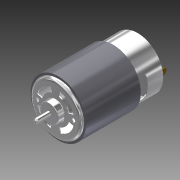
# Autodesk Inventor part: RS-550
Saved by Autodesk Inventor 2015 SP1 (Build 190203100, 203)
## iProperties
Category: Motors
Company: Autodesk, Inc.
Shininess: 64.0
Length Units: 11269
Angle Units: 11279
Time Units: 11290
Mass Units: 11283
Length Display Precision: 3
Angle Display Precision: 2
Compacted: True
Part Number: RS-550
Document SubType Name: Modeling
Created: 2014-12-12
Material: Steel, Mild
Project: FIRST
Catalog Web Link: http://banebots.com/pc/p/M5-RS550-12
Vendor: BaneBots
Density: 40.6947 g/cm^3
Description: Motor - BaneBots RS-550
Mass: 221 g
Surface Area: 167.862 cm^2
Volume: 12.5148 cm^3
Appearance: Chrome - Polished
Density: 0.0
Volumn: 0.0
Area: 0.0
PropertySet Name: Model Information
Control State: 0
Master: False
Checked Out: False
Title: Motor - BaneBots RS-550
Author: Autodesk, Inc.
Autodesk Inventor part; units mm, degrees
sketch "Sketch1" plane through (0, 0, 0) normal (0, 0, 1) x (1, 0, 0)
  circle A0 centre (0, 0) radius 17.75
  dimension "d0" = 35.5
  constraints: 2 coincident, 1 centre point, 2 other
  measures "d0" diameter of A0
extrude "Extrusion1" add sketch "Sketch1" along normal mid plane 57
fillet "Fillet1" radius 2 1 edges at (-17.75, 0, 28.5)
shell "Shell1" thickness 0.62 removed faces 1 at (3.0438, 4.2648, -28.5)
sketch "Sketch2" plane through (0, 0, 28.5) normal (0, 0, 1) x (1, 0, 0)
  circle A0 centre (0, 0) radius 15.75 projected
  circle A1 centre (0, 0) radius 6.5
  dimension "d5" = 13
  constraints: 1 centre point, 1 coincident, 1 concentric
  measures "d5" diameter of A1
extrude "Extrusion2" add sketch "Sketch2" along normal blind 4.5 contours A1
fillet "Fillet2" radius 0.5 2 edges at (-6.5, 0, 28.5) (-6.5, 0, 33)
sketch "Sketch3" plane through (0, 0, 33) normal (0, 0, 1) x (1, 0, 0)
  circle A0 centre (0, 0) radius 6 projected
  circle A1 centre (0, 0) radius 1.6
  dimension "d9" = 3.2
  constraints: 1 centre point, 1 coincident, 1 concentric
  measures "d9" diameter of A1
extrude "Extrusion3" add sketch "Sketch3" along normal blind 10 contours A1
fillet "Fillet3" radius 1.6 1 edges at (-1.6, 0, 43)
sketch "Sketch4" plane through (0, 0, 28.5) normal (0, 0, 1) x (1, 0, 0)
  circle A0 centre (0, 0) radius 15.75 projected
  point P0 (12.5, 0)
  dimension "d13" = 12.5
  constraints: 1 horizontal alignment
  measures "d13" distance of point (12.5, 0) A0.centre
hole "Hole1" at (12.5, 0, 28.5) direction (0, 0, -1) diameter 2.5 depth 8 tip angle 118
mirror "Mirror1" about plane through (0, 0, 0) normal (1, 0, 0) of "Hole1"
sketch "Sketch5" plane through (0, 0, 28.5) normal (0, 0, 1) x (1, 0, 0)
  circle A0 centre (12.5, 0) radius 1.25 projected
  circle A1 centre (0, 0) radius 7 projected
  arc A2 (12.557, 3.3646) -> (3.3646, 12.557) centre (0, 0) ccw
  arc A3 (9.1763, 2.4588) -> (2.4588, 9.1763) centre (0, 0) ccw
  line L0 (0, 0) -> (3.3646, 12.557) construction
  line L1 (0, 0) -> (12.557, 3.3646) construction
  line L2 (2.4588, 9.1763) -> (3.3646, 12.557)
  line L3 (9.1763, 2.4588) -> (12.557, 3.3646)
  line L4 (0, 0) -> (12.5, 0) construction
  line L5 (0.151, 0.5634) -> (0.151, 14.7153) construction
  dimension "d21" = 15
  dimension "d22" = 15
  dimension "d23" = 13
  dimension "d24" = 9.5
  constraints: 12 end point, 4 point on circle, 3 point on line, 2 centre point, 2 coincident, 2 collinear, 2 concentric, 1 horizontal, 1 perpendicular
  measures "d21" angle of L1 L4
  measures "d22" angle of L5 L0
  measures "d23" radius of A2
  measures "d24" radius of A3
extrude "Extrusion4" cut sketch "Sketch5" against normal blind 10 contours L3 A3 L2 A2
pattern_circular "Circular Pattern1" count 4 over 360 about axis through (0, 0, 0) along (0, 0, 1) of "Extrusion4"
ref_plane "Work Plane1" through (0, 0, -26.75) normal (0, 0, -1) x (-1, 0, 0)
sketch "Sketch6" plane through (0, 0, -26.75) normal (0, 0, -1) x (-1, 0, 0)
  circle A0 centre (0, 0) radius 17.13 projected
extrude "Extrusion5" add sketch "Sketch6" against normal blind 0.62
sketch "Sketch7" plane through (0, 0, -26.75) normal (0, 0, -1) x (-1, 0, 0)
  circle A0 centre (0, 0) radius 17.13 projected
  circle A1 centre (0, 0) radius 12
  dimension "d33" = 24
  constraints: 1 centre point, 1 coincident, 1 concentric
  measures "d33" diameter of A1
extrude "Extrusion6" add sketch "Sketch7" along normal blind 0.62 contours A1
sketch "Sketch8" plane through (0, 0, -27.37) normal (0, 0, -1) x (-1, 0, 0)
  circle A0 centre (0, 0) radius 12 projected
  circle A1 centre (0, 0) radius 5.375
  dimension "d36" = 10.75
  constraints: 1 centre point, 1 coincident, 1 concentric
  measures "d36" diameter of A1
extrude "Extrusion7" add sketch "Sketch8" along normal blind 3 contours A1
sketch "Sketch9" plane through (0, 0, -30.37) normal (0, 0, -1) x (-1, 0, 0)
  circle A0 centre (0, 0) radius 5.375 projected
  circle A1 centre (0, 0) radius 3.45
  dimension "d39" = 6.9
  constraints: 1 centre point, 1 coincident, 1 concentric
  measures "d39" diameter of A1
extrude "Extrusion8" cut sketch "Sketch9" against normal blind 0.8 contours A1
sketch "Sketch10" plane through (0, 0, -29.57) normal (0, 0, -1) x (-1, 0, 0)
  circle A0 centre (0, 0) radius 3.45 projected
  circle A1 centre (0, 0) radius 1.6
  dimension "d42" = 3.2
  constraints: 1 centre point, 1 coincident, 1 concentric
  measures "d42" diameter of A1
extrude "Extrusion9" add sketch "Sketch10" along normal blind 1 contours A1
sketch "Sketch11" plane through (0, 0, -27.37) normal (0, 0, -1) x (-1, 0, 0)
  circle A0 centre (0, 0) radius 5.375 projected
  circle A1 centre (0, 0) radius 12 projected
  arc A2 (9.3591, 3.15) -> (3.15, 9.3591) centre (0, 0) ccw
  arc A3 (5.6857, 3.15) -> (3.15, 5.6857) centre (0, 0) ccw
  line L0 (3.15, 9.3591) -> (3.15, 5.6857)
  line L1 (5.6857, 3.15) -> (9.3591, 3.15)
  dimension "d45" = 3.15
  dimension "d46" = 3.15
  dimension "d47" = 9.875
  dimension "d48" = 6.5
  constraints: 4 end point, 4 point on circle, 2 centre point, 2 coincident, 2 concentric, 1 perpendicular, 1 vertical
  measures "d45" distance from line of L0 A3.centre
  measures "d46" distance from line of A0.centre L1
  measures "d47" radius of A2
  measures "d48" radius of A3
extrude "Extrusion10" cut sketch "Sketch11" against normal blind 1 contours L1 A3 L0 A2
pattern_circular "Circular Pattern2" count 4 over 360 about axis through (0, 0, 0) along (0, 0, 1) of "Extrusion10"
sketch "Sketch12" plane through (0, 0, -26.75) normal (0, 0, -1) x (-1, 0, 0)
  circle A0 centre (0, 0) radius 12 projected
  circle A1 centre (0, 0) radius 17.13 projected
  line L0 (-14.5, 1.9) -> (-14, 1.9)
  line L1 (-14, 1.9) -> (-14, -1.9)
  line L2 (-14, -1.9) -> (-14.5, -1.9)
  line L3 (-14.5, -1.9) -> (-14.5, 1.9)
  line L4 (0, 0) -> (-16.9017, 0) construction
  point P0 (-14, 0)
  dimension "d54" = 0.5
  dimension "d55" = 3.8
  dimension "d56" = 14
  constraints: 10 end point, 2 parallel, 2 perpendicular, 1 horizontal, 1 midpoint, 1 point on line
  measures "d54" distance of L1.end L2.end
  measures "d55" distance of L2.end L0.start
  measures "d56" distance from line of L1 A0.centre
extrude "Extrusion11" add sketch "Sketch12" along normal blind 7.2 contours L0 L1 L2 L3
chamfer "Chamfer1" distance 1 angle 45 2 edges at (14.25, 1.9, -33.95) (14.25, -1.9, -33.95)
sketch "Sketch13" plane through (14.5, -1.9, -26.75) normal (1, 0, 0) x (0, 0, -1)
  line L0 (7.2, 1) -> (7.2, 2.8) projected
  line L1 (4.2, 1.9) -> (6.2, 3.8) construction
  line L2 (4.2, 1.9) -> (6.2, 0) construction
  dimension "d61" = 3
  constraints: 4 end point, 1 equal length
  measures "d61" distance from line of L0 L1.start
hole "Hole2" at (14.5, 0, -30.95) direction (-1, 0, 0) diameter 2 depth 1 tip angle 118
mirror "Mirror2" about plane through (0, 0, 0) normal (1, 0, 0) of "Extrusion11", "Chamfer1", "Hole2"
ref_plane "Work Plane2" through (18, 0, 0) normal (1, 0, 0) x (0, 1, 0)
sketch "Sketch14" plane through (18, 0, 0) normal (1, 0, 0) x (0, 1, 0)
  arc A0 (-4.5554, -11.85) -> (-4.5554, -17.75) centre (-4.5554, -14.8) ccw
  arc A1 (5.2946, -17.75) -> (5.2946, -11.85) centre (5.2946, -14.8) ccw
  line L0 (-4.5554, -11.85) -> (5.2946, -11.85)
  line L1 (-4.5554, -17.75) -> (5.2946, -17.75)
  line L2 (17.75, -28.5) -> (-17.75, -28.5) projected
  line L3 (0, -28.5) -> (0, 17.1564) construction
  dimension "d70" = 10.75
  dimension "d71" = 5.9
  dimension "d72" = 9.85
  constraints: 6 end point, 4 point on circle, 4 tangent, 2 centre point, 1 equal radius, 1 horizontal, 1 horizontal alignment, 1 midpoint, 1 parallel, 1 perpendicular
  measures "d70" distance between parallel lines of L2 L1
  measures "d71" distance between parallel lines of L0 L1
  measures "d72" distance of A1.centre A0.centre
extrude "Extrusion12" cut sketch "Sketch14" against normal through all
ref_plane "Work Plane3" through (0, 0, 26.5) normal (0, 0, -1) x (-1, 0, 0)
sketch "Sketch15" plane through (0, 0, 26.5) normal (0, 0, -1) x (-1, 0, 0)
  circle A0 centre (0, 0) radius 17.75 projected
  circle A1 centre (0, 0) radius 19.25
  dimension "d76" = 1.5
  constraints: 1 centre point
  measures "d76" radial gap between concentric circles of A1 A0
extrude "Flux Ring" add sketch "Sketch15" along normal blind 38
body "Solid1"
